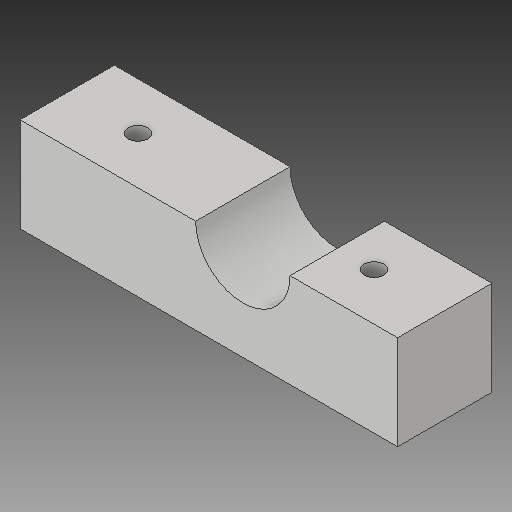
# Autodesk Inventor part: HoldWormDrive
Saved by Autodesk Inventor 2019.3 (Build 233278000, 278)
## iProperties
Created: 2019-01-19
Part Number: HoldWormDrive
Material: Generic
Document SubType Name: Modeling
Designer: steele
Density: 1 g/cm^3
Appearance: Default
Author: steele
Autodesk Inventor part; units mm, degrees
ref_plane "YZ Plane" through (0, 0, 0) normal (1, 0, 0) x (0, 1, 0)
ref_plane "XZ Plane" through (0, 0, 0) normal (0, 1, 0) x (-1, 0, 0)
ref_plane "XY Plane" through (0, 0, 0) normal (0, 0, 1) x (1, 0, 0)
sketch "Sketch1" plane through (0, 0, 0) normal (0, 1, 0) x (-1, 0, 0)
  line L0 (25.4, 6.35) -> (-25.4, 6.35)
  line L1 (-25.4, 6.35) -> (-25.4, -6.35)
  line L2 (-25.4, -6.35) -> (25.4, -6.35)
  line L3 (25.4, -6.35) -> (25.4, 6.35)
  line L4 (25.4, 6.35) -> (-25.4, -6.35) construction
  line L5 (-25.4, 6.35) -> (25.4, -6.35) construction
  point P0 (0, 0)
  dimension "d0" = 50.8
  dimension "d1" = 12.7
  constraints: 12 end point, 2 midpoint, 2 parallel, 1 horizontal, 1 perpendicular
  measures "d0" distance of L0.start L0.end
  measures "d1" distance of L1.end L0.end
extrude "Extrusion1" add sketch "Sketch1" against normal blind 12.7
sketch "Sketch3" plane through (-25.4, 0, 6.35) normal (0, 0, 1) x (1, 0, 0)
  line L0 (0, 0) -> (50.8, 0) projected
  line L1 (0, 0) -> (0, -12.7) projected
  line L2 (50.8, -12.7) -> (0, -12.7) projected
  line L3 (50.8, 0) -> (50.8, -12.7) projected
  circle A0 centre (29.981, 0) radius 6.35 projected
  point P0 (25.4, 0)
extrude "Extrusion2" cut sketch "Sketch3" against normal through all contours A0 L0 | L0 A0
sketch "Sketch4" plane through (0, -12.7, 0) normal (0, -1, 0) x (1, 0, 0)
  line L0 (-25.4, 6.35) -> (-25.4, -6.35) construction
  line L1 (-25.4, 0) -> (25.4, 0) construction
  line L2 (25.4, -6.35) -> (25.4, 6.35) construction
  point P0 (0, 0)
  point P1 (-15.875, 0)
  point P2 (15.875, 0)
  dimension "d6" = 9.525
  dimension "d7" = 9.525
  constraints: 2 end point, 2 midpoint, 2 point on line
  measures "d6" distance from line of point (-15.875, 0) L0
  measures "d7" distance from line of point (15.875, 0) L2
hole "Hole1" at (-15.875, -12.7, 0) at (15.875, -12.7, 0) direction (0, 1, 0) diameter 2.6416 end through all thread size "6-32 UNC" class "2B" standard "ANSI Unified Screw Threads"
sketch "Sketch7" plane through (0, -12.7, 0) normal (0, -1, 0) x (1, 0, 0)
  circle A0 centre (-15.875, 0) radius 1.3208 projected
  circle A1 centre (-15.875, 0) radius 2.4257
  circle A2 centre (15.875, 0) radius 1.3208 projected
  circle A3 centre (15.875, 0) radius 2.4257
  point P0 (0, 0)
  dimension "d18" = 4.8514
  constraints: 2 centre point, 2 coincident, 1 equal radius
  measures "d18" diameter of A1
extrude "Extrusion4" cut sketch "Sketch7" against normal blind 7.1374
body "Solid1"
